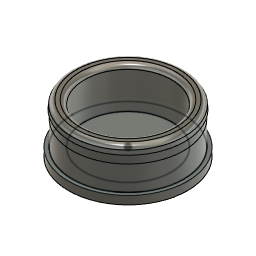
Empty+I_O (Autodesk Fusion 360 design; units mm, degrees)
Autodesk Fusion 360 part; units mm, degrees
sketch "Esboço1" plane through (0, 0, 0) normal (0, 1, 0) x (1, 0, 0)
  circle A0 centre (0, 0) radius 7.25
  dimension "d1" = 14.5
  constraint coincident A0.centre origin
  measures "d1" diameter of A0
extrude "Extrusão1" add sketch "Esboço1" along normal blind 1
sketch "Esboço2" plane through (0, 1, 0) normal (0, 1, 0) x (-1, 0, 0)
  circle A0 centre (0, 0) radius 7.25
  circle A1 centre (0, 0) radius 6.8
  circle A2 centre (0, 0) radius 5.3
  dimension "d4" = 13.6
  dimension "d5" = -1.5
  constraint concentric A0 A1
  measures "d4" diameter of A1
extrude "Extrusão2" add sketch "Esboço2" along normal blind 5 contours A1
sketch "Esboço3" plane through (0, 0, 0) normal (0, 0, 1) x (1, 0, 0)
  line L0 (6.8, 6) -> (6.8, 4)
  line L1 (6.8, 5) -> (6.9, 5)
  line L2 (6.9, 5) -> (6.8, 4)
  line L3 (6.9, 5) -> (6.8, 6)
  constraint vertical L0
  constraint midpoint L0 L1.start
  constraint perpendicular L0 L1
revolve "Revolucionar1" add sketch "Esboço3" angle 360 about axis through (0, 1.75, 0) along (0, 1, 0)
fillet "Arredondamento1" radius 0.55 1 edges at (6.3398, 6, -2.459)
fillet "Arredondamento2" radius 0.55 1 edges at (4.9413, 6, 1.9166)
